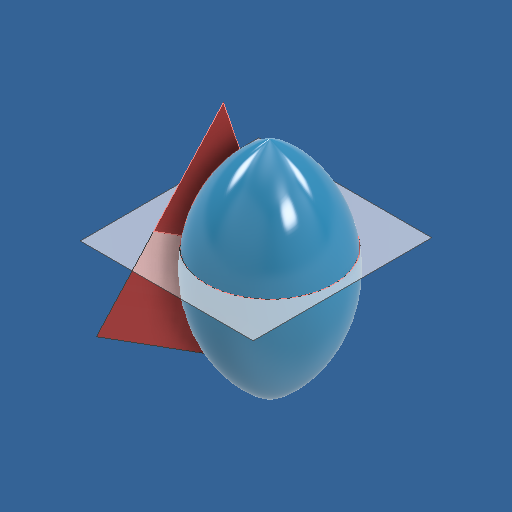
# Autodesk Inventor part: идз3
Saved by Autodesk Inventor 2025 (Build 290162000, 162)
## iProperties
Created: 2024-11-13
Part Number: идз3
Material: Типовые
Document SubType Name: Modeling
Designer: Asus
Density: 1 g/cm^3
Appearance: По умолчанию
Author: Asus
Autodesk Inventor part; units mm, degrees
ref_plane "YZ Plane" through (0, 0, 0) normal (1, 0, 0) x (0, 1, 0)
ref_plane "XY Plane" through (0, 0, 0) normal (0, 0, 1) x (1, 0, 0)
sketch "Эскиз1" plane through (0, 0, 0) normal (0, 1, 0) x (-1, 0, 0)
  line L0 (25, -43.3013) -> (25, 43.3013)
  line L1 (25, 43.3013) -> (-50, 0)
  line L2 (25, -43.3013) -> (-50, 0)
  point P0 (0, 0)
  constraints: 6 end point
sketch "Эскиз3" plane through (0, 0, 0) normal (0, 0, 1) x (1, 0, 0)
  line L0 (-25, 0) -> (50, 0) projected
  line L1 (50, 0) -> (0, 100) construction
  point P0 (0, 0)
  constraints: 2 end point
loft "Лофт1" add profiles "Эскиз1" section 2 point at (0, 100, 0)
sketch "Эскиз4" plane through (0, 0, 0) normal (0, 0, 1) x (1, 0, 0)
  line L0 (50, 0) -> (-25, 0) projected
  arc A0 (25, 95.6218) -> (25, -25.6218) centre (60, 35) ccw
  line L1 (25, -25.6218) -> (25, 95.6218)
  point P0 (0, 0)
  dimension "d12" = 140
  constraints: 2 end point, 2 point on circle, 1 centre point, 1 vertical
  measures "d12" diameter of A0
revolve "Вращение1" add sketch "Эскиз4" angle 360 about axis through (25, -25.6218, 0) along (0, 1, 0)
ref_plane "РабПлоскость1" through (0, 45, 0) normal (0, 1, 0) x (-1, 0, 0)
split body "Разделение1" result two bodies by plane through (0, 45, 0) normal (0, 1, 0) first body at (0.037, 50.5291, -21.1883)
sketch "Эскиз5" plane through (0, 45, 0) normal (0, 1, 0) x (-1, 0, 0)
  line L0 (29, -48) -> (-64, -48)
  line L1 (-64, -48) -> (-64, 48)
  line L2 (-64, 48) -> (29, 48)
  line L3 (29, 48) -> (29, -48)
  point P0 (0, 0)
  constraints: 8 end point, 2 parallel, 1 horizontal, 1 perpendicular
extrude "Выдавливание1" add sketch "Эскиз5" against normal blind 0.1 separate body
